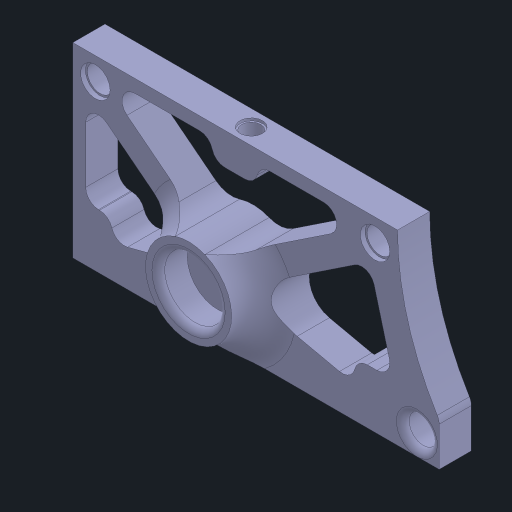
# Autodesk Inventor part: gear_holder_r
Saved by Autodesk Inventor 2023 (Build 270158000, 158)
## iProperties
Created: 2024-06-01
Part Number: gear_holder_r
Material: ABS Plastic
Document SubType Name: Modeling
Designer: szymo
Density: 1.06 g/cm^3
Appearance: Slate Blue
Mass: 5.35805 g
Surface Area: 42.0736 cm^2
Volume: 5.05477 cm^3
TOTAL MASS: 0.0
Author: szymo
Autodesk Inventor part; units mm, degrees
ref_plane "YZ Plane" through (0, 0, 0) normal (1, 0, 0) x (0, 1, 0)
ref_plane "XZ Plane" through (0, 0, 0) normal (0, 1, 0) x (-1, 0, 0)
ref_plane "XY Plane" through (0, 0, 0) normal (0, 0, 1) x (1, 0, 0)
sketch "Sketch10" plane through (0, 0, 0) normal (0, 0, 1) x (1, 0, 0)
  circle A0 centre (29.9359, 0.3357) radius 2 projected
  circle A1 centre (-0.5678, 6.6482) radius 4.5 projected
  circle A2 centre (41.9322, 11.1482) radius 15 projected
  line L0 (99.4322, -2.8518) -> (37.7886, -2.8518) projected
  line L1 (-23.5678, -2.8518) -> (-23.5678, 26.1482) projected
  circle A3 centre (-0.5678, 6.6482) radius 4.575
  circle A4 centre (-0.5678, 6.6482) radius 5.975
  circle A5 centre (29.9359, 0.3357) radius 2.075
  circle A6 centre (29.9359, 0.3357) radius 3.475
  line L2 (22.0831, -2.8518) -> (-23.5678, -2.8518) projected
  line L3 (28.5518, -2.8518) -> (22.0831, -2.8518) projected
  line L4 (31.32, -2.8518) -> (28.5518, -2.8518) projected
  line L5 (37.7886, -2.8518) -> (31.32, -2.8518) projected
  line L6 (-23.5678, 26.1482) -> (111.997, 26.1482) projected
  line L7 (-23.5678, 26.1482) -> (26.9322, 26.1482)
  line L8 (26.9322, 26.1482) -> (26.9322, -2.8518)
  line L9 (26.9322, -2.8518) -> (-23.5678, -2.8518)
  line L10 (-23.5678, -2.8518) -> (-23.5678, 26.1482)
  line L11 (26.9322, 26.1482) -> (19.9322, 26.1482)
  line L12 (19.9322, 26.1482) -> (19.9322, 19.1482)
  line L13 (19.9322, 19.1482) -> (26.9322, 19.1482)
  line L14 (26.9322, 19.1482) -> (26.9322, 26.1482)
  line L15 (-23.5678, 26.1482) -> (-16.5678, 26.1482)
  line L16 (-16.5678, 26.1482) -> (-16.5678, 19.1482)
  line L17 (-16.5678, 19.1482) -> (-23.5678, 19.1482)
  line L18 (-23.5678, 19.1482) -> (-23.5678, 26.1482)
  line L19 (-23.5678, -2.8518) -> (-17.5678, -2.8518)
  line L20 (-17.5678, -2.8518) -> (-17.5678, 5.1482)
  line L21 (-17.5678, 5.1482) -> (-23.5678, 5.1482)
  line L22 (-23.5678, 5.1482) -> (-23.5678, -2.8518)
  line L23 (26.4609, -2.8518) -> (20.4609, -2.8518)
  line L24 (20.4609, -2.8518) -> (20.4609, 5.1482)
  line L25 (20.4609, 5.1482) -> (26.4609, 5.1482)
  line L26 (26.4609, 5.1482) -> (26.4609, -2.8518)
  line L27 (26.9322, -2.8518) -> (33.4109, -2.8518)
  line L28 (33.4109, -2.8518) -> (33.4109, 3.8107)
  line L29 (33.4109, 3.8107) -> (26.9322, 3.8107)
  line L30 (26.9322, 3.8107) -> (26.9322, -2.8518)
  line L31 (26.9322, 26.1482) -> (33.4109, 3.8107)
  circle A7 centre (68.6798, 26.1482) radius 41.7476
  point P0 (0, 0)
  point P1 (28.9333, 3.6629)
  point P2 (28.8494, 3.8107)
  point P3 (29.9359, 3.8107)
  point P4 (38.6488, -2.8518)
  point P5 (26.9322, 26.1482)
  dimension "d122" = 0.075
  dimension "d123" = 1.4
  dimension "d124" = 0.075
  dimension "d125" = 1.4
  dimension "d126" = 7
  dimension "d127" = 7
  dimension "d128" = 7
  dimension "d129" = 7
  dimension "d130" = 6
  dimension "d131" = 8
  dimension "d132" = 6
  dimension "d133" = 8
  constraints: 50 end point, 12 parallel, 6 horizontal, 6 perpendicular, 4 centre point, 4 tangent, 3 point on line, 1 vertical, 3 other
  measures "d122" radial gap between concentric circles of A1 A3
  measures "d123" radial gap between concentric circles of A3 A4
  measures "d124" radial gap between concentric circles of A0 A5
  measures "d125" radial gap between concentric circles of A5 A6
  measures "d126" distance of L13.end L12.end
  measures "d127" distance of L12.end L11.end
  measures "d128" distance of L16.end L17.end
  measures "d129" distance of L15.end L16.end
  measures "d130" distance of L21.end L20.end
  measures "d131" distance of L20.end L19.end
  measures "d132" distance of L24.end L25.end
  measures "d133" distance of L23.end L24.end
extrude "bryla" add sketch "Sketch10" along normal blind 5 contours A0 A2 | A0 A2 A5 | A2 A0 | A0 A2 A5 | A5 A2 A6 L4 L8 | A2 A6 A5 | A6 L8 L29 A2 | A2 L29 A6 | A6 L28 A2 | A2 L28 L5 A6 | L29 L8 A2 | A2 A7 L29 | L29 L28 A6 | L8 A6 | A6 L26 L25 L24 L2 L20 L21 L1 L17 L16 L6 L12 L13 L8 | L8 A7 A2 | L26 L3 L2 L24 L25 | A6 L8 L3 L26 | A6 L3 L8 | L13 L12 L6 L8 | L16 L17 L1 L6 | L2 L1 L21 L20 | A1 | A3 | A4
sketch "Sketch11" plane through (0, 0, 5) normal (0, 0, 1) x (1, 0, 0)
  circle A0 centre (29.9359, 0.3357) radius 2 projected
  arc A1 (29.2892, -11.6469) -> (30.1063, -9.4128) centre (21.6078, -7.5708) ccw projected
  arc A2 (30.1063, -9.4128) -> (30.8013, -9.3758) centre (29.9359, 0.3357) ccw projected
  arc A3 (30.8013, -9.3758) -> (31.851, -11.5105) centre (39.0563, -6.642) ccw projected
  arc A4 (31.851, -11.5105) -> (32.6912, -11.3437) centre (29.9359, 0.3357) ccw projected
  arc A5 (32.6912, -11.3437) -> (32.8459, -8.9699) centre (24.1726, -9.5968) ccw projected
  arc A6 (32.8459, -8.9699) -> (33.5023, -8.7386) centre (29.9359, 0.3357) ccw projected
  arc A7 (33.5023, -8.7386) -> (35.1109, -10.4911) centre (40.6527, -3.7898) ccw projected
  arc A8 (35.1109, -10.4911) -> (35.8701, -10.0943) centre (29.9359, 0.3357) ccw projected
  arc A9 (35.8701, -10.0943) -> (35.3497, -7.7731) centre (27.2044, -10.8182) ccw projected
  arc A10 (35.3497, -7.7731) -> (35.9144, -7.3662) centre (29.9359, 0.3357) ccw projected
  arc A11 (35.9144, -7.3662) -> (37.9515, -8.5945) centre (41.3809, -0.6035) ccw projected
  arc A12 (37.9515, -8.5945) -> (38.5682, -8) centre (29.9359, 0.3357) ccw projected
  arc A13 (38.5682, -8) -> (37.4149, -5.9194) centre (30.4575, -11.1359) ccw projected
  arc A14 (37.4149, -5.9194) -> (37.8421, -5.3699) centre (29.9359, 0.3357) ccw projected
  arc A15 (37.8421, -5.3699) -> (40.1428, -5.9745) centre (41.1819, 2.659) ccw projected
  arc A16 (40.1428, -5.9745) -> (40.5669, -5.2303) centre (29.9359, 0.3357) ccw projected
  arc A17 (40.5669, -5.2303) -> (38.8742, -3.5589) centre (33.6683, -10.5243) ccw projected
  arc A18 (38.8742, -3.5589) -> (39.1293, -2.9114) centre (29.9359, 0.3357) ccw projected
  arc A19 (39.1293, -2.9114) -> (41.5071, -2.8433) centre (40.0718, 5.7333) ccw projected
  arc A20 (41.5071, -2.8433) -> (41.7044, -2.0097) centre (29.9359, 0.3357) ccw projected
  arc A21 (41.7044, -2.0097) -> (39.6094, -0.883) centre (36.5767, -9.0328) ccw projected
  arc A22 (39.6094, -0.883) -> (39.6717, -0.1898) centre (29.9359, 0.3357) ccw projected
  arc A23 (39.6717, -0.1898) -> (41.934, 0.5455) centre (38.1405, 8.3702) ccw projected
  arc A24 (41.934, 0.5455) -> (41.8885, 1.4009) centre (29.9359, 0.3357) ccw projected
  arc A25 (41.8885, 1.4009) -> (39.5609, 1.8918) centre (38.9471, -6.7824) ccw projected
  arc A26 (39.5609, 1.8918) -> (39.4254, 2.5744) centre (29.9359, 0.3357) ccw projected
  arc A27 (39.4254, 2.5744) -> (41.3889, 3.9172) centre (35.5446, 10.3563) ccw projected
  arc A28 (41.3889, 3.9172) -> (41.1043, 4.7252) centre (29.9359, 0.3357) ccw projected
  arc A29 (41.1043, 4.7252) -> (38.7326, 4.5404) centre (40.5875, -3.9553) ccw projected
  arc A30 (38.7326, 4.5404) -> (38.4103, 5.1572) centre (29.9359, 0.3357) ccw projected
  arc A31 (38.4103, 5.1572) -> (39.916, 6.9989) centre (32.4943, 11.5305) ccw projected
  arc A32 (39.916, 6.9989) -> (39.4152, 7.6939) centre (29.9359, 0.3357) ccw projected
  arc A33 (39.4152, 7.6939) -> (37.1917, 6.8484) centre (41.3649, -0.7806) ccw projected
  arc A34 (37.1917, 6.8484) -> (36.7086, 7.3495) centre (29.9359, 0.3357) ccw projected
  arc A35 (36.7086, 7.3495) -> (37.6345, 9.5407) centre (29.2367, 11.7979) ccw projected
  arc A36 (37.6345, 9.5407) -> (36.9582, 10.0664) centre (29.9359, 0.3357) ccw projected
  arc A37 (36.9582, 10.0664) -> (35.063, 8.6288) centre (41.2165, 2.4846) ccw projected
  arc A38 (35.063, 8.6288) -> (34.4583, 8.9734) centre (29.9359, 0.3357) ccw projected
  arc A39 (34.4583, 8.9734) -> (34.7293, 11.3368) centre (26.0358, 11.1366) ccw projected
  arc A40 (34.7293, 11.3368) -> (33.9323, 11.6507) centre (29.9359, 0.3357) ccw projected
  arc A41 (33.9323, 11.6507) -> (32.5188, 9.7373) centre (40.1541, 5.5756) ccw projected
  arc A42 (32.5188, 9.7373) -> (31.8415, 9.8977) centre (29.9359, 0.3357) ccw projected
  arc A43 (31.8415, 9.8977) -> (31.4358, 12.2416) centre (23.1508, 9.6003) ccw projected
  arc A44 (31.4358, 12.2416) -> (30.5826, 12.3183) centre (29.9359, 0.3357) ccw projected
  arc A45 (30.5826, 12.3183) -> (29.7655, 10.0842) centre (38.264, 8.2422) ccw projected
  arc A46 (29.7655, 10.0842) -> (29.0704, 10.0472) centre (29.9359, 0.3357) ccw projected
  arc A47 (29.0704, 10.0472) -> (28.0208, 12.1819) centre (20.8155, 7.3134) ccw projected
  arc A48 (28.0208, 12.1819) -> (27.1805, 12.0151) centre (29.9359, 0.3357) ccw projected
  arc A49 (27.1805, 12.0151) -> (27.0259, 9.6413) centre (35.6991, 10.2682) ccw projected
  arc A50 (27.0259, 9.6413) -> (26.3695, 9.41) centre (29.9359, 0.3357) ccw projected
  arc A51 (26.3695, 9.41) -> (24.7609, 11.1625) centre (19.2191, 4.4613) ccw projected
  arc A52 (24.7609, 11.1625) -> (24.0017, 10.7657) centre (29.9359, 0.3357) ccw projected
  arc A53 (24.0017, 10.7657) -> (24.5221, 8.4445) centre (32.6674, 11.4896) ccw projected
  arc A54 (24.5221, 8.4445) -> (23.9574, 8.0377) centre (29.9359, 0.3357) ccw projected
  arc A55 (23.9574, 8.0377) -> (21.9202, 9.266) centre (18.4909, 1.2749) ccw projected
  arc A56 (21.9202, 9.266) -> (21.3036, 8.6714) centre (29.9359, 0.3357) ccw projected
  arc A57 (21.3036, 8.6714) -> (22.4568, 6.5908) centre (29.4143, 11.8073) ccw projected
  arc A58 (22.4568, 6.5908) -> (22.0297, 6.0413) centre (29.9359, 0.3357) ccw projected
  arc A59 (22.0297, 6.0413) -> (19.729, 6.646) centre (18.6899, -1.9876) ccw projected
  arc A60 (19.729, 6.646) -> (19.3048, 5.9017) centre (29.9359, 0.3357) ccw projected
  arc A61 (19.3048, 5.9017) -> (20.9975, 4.2304) centre (26.2035, 11.1957) ccw projected
  arc A62 (20.9975, 4.2304) -> (20.7425, 3.5828) centre (29.9359, 0.3357) ccw projected
  arc A63 (20.7425, 3.5828) -> (18.3646, 3.5147) centre (19.8, -5.0618) ccw projected
  arc A64 (18.3646, 3.5147) -> (18.1673, 2.6811) centre (29.9359, 0.3357) ccw projected
  arc A65 (18.1673, 2.6811) -> (20.2623, 1.5544) centre (23.2951, 9.7043) ccw projected
  arc A66 (20.2623, 1.5544) -> (20.2001, 0.8612) centre (29.9359, 0.3357) ccw projected
  arc A67 (20.2001, 0.8612) -> (17.9377, 0.126) centre (21.7312, -7.6988) ccw projected
  arc A68 (17.9377, 0.126) -> (17.9832, -0.7294) centre (29.9359, 0.3357) ccw projected
  arc A69 (17.9832, -0.7294) -> (20.3108, -1.2203) centre (20.9247, 7.4538) ccw projected
  arc A70 (20.3108, -1.2203) -> (20.4464, -1.903) centre (29.9359, 0.3357) ccw projected
  arc A71 (20.4464, -1.903) -> (18.4828, -3.2458) centre (24.3272, -9.6849) ccw projected
  arc A72 (18.4828, -3.2458) -> (18.7675, -4.0537) centre (29.9359, 0.3357) ccw projected
  arc A73 (18.7675, -4.0537) -> (21.1391, -3.869) centre (19.2843, 4.6267) ccw projected
  arc A74 (21.1391, -3.869) -> (21.4615, -4.4858) centre (29.9359, 0.3357) ccw projected
  arc A75 (21.4615, -4.4858) -> (19.9558, -6.3274) centre (27.3775, -10.8591) ccw projected
  arc A76 (19.9558, -6.3274) -> (20.4566, -7.0224) centre (29.9359, 0.3357) ccw projected
  arc A77 (20.4566, -7.0224) -> (22.6801, -6.177) centre (18.5068, 1.452) ccw projected
  arc A78 (22.6801, -6.177) -> (23.1631, -6.678) centre (29.9359, 0.3357) ccw projected
  arc A79 (23.1631, -6.678) -> (22.2373, -8.8693) centre (30.6351, -11.1264) ccw projected
  arc A80 (22.2373, -8.8693) -> (22.9136, -9.395) centre (29.9359, 0.3357) ccw projected
  arc A81 (22.9136, -9.395) -> (24.8088, -7.9574) centre (18.6553, -1.8131) ccw projected
  arc A82 (24.8088, -7.9574) -> (25.4135, -8.302) centre (29.9359, 0.3357) ccw projected
  arc A83 (25.4135, -8.302) -> (25.1425, -10.6653) centre (33.836, -10.4652) ccw projected
  arc A84 (25.1425, -10.6653) -> (25.9395, -10.9793) centre (29.9359, 0.3357) ccw projected
  arc A85 (25.9395, -10.9793) -> (27.3529, -9.0659) centre (19.7176, -4.9042) ccw projected
  arc A86 (27.3529, -9.0659) -> (28.0302, -9.2262) centre (29.9359, 0.3357) ccw projected
  arc A87 (28.0302, -9.2262) -> (28.436, -11.5702) centre (36.721, -8.9289) ccw projected
  arc A88 (28.436, -11.5702) -> (29.2892, -11.6469) centre (29.9359, 0.3357) ccw projected
  line L0 (-23.5678, -2.8518) -> (33.4109, -2.8518) projected
  circle A89 centre (29.9359, 0.3357) radius 2.2
  circle A90 centre (29.9359, 0.3357) radius 4.2
  point P0 (0, 0)
  dimension "d136" = 0.2
  dimension "d137" = 2
  constraints: 2 centre point
  measures "d136" radial gap between concentric circles of A0 A89
  measures "d137" radial gap between concentric circles of A89 A90
extrude "smolZebatkaDziura" cut sketch "Sketch11" against normal blind 4 contours A0 | A89
sketch "Sketch12" plane through (0, 0, 5) normal (0, 0, 1) x (1, 0, 0)
  circle A0 centre (-0.5678, 6.6482) radius 4.5 projected
  circle A1 centre (-0.5678, 6.6482) radius 4.7
  point P0 (0, 0)
  dimension "d202" = 0.2
  constraints: 1 centre point
  measures "d202" radial gap between concentric circles of A0 A1
ref_plane "Work Plane4" through (-6.5573, 0.6587, 5.5) normal (0, 0, -1) x (0.4265437, 0.9044669, 0)
extrude "duzaZebatkPodpora" add sketch "Sketch12" along normal up to surface (0.5 mm away) contours A0 | A1
sketch "Sketch13" plane through (0, 0, 5) normal (0, 0, 1) x (1, 0, 0)
  circle A0 centre (-0.5678, 6.6482) radius 4.5 projected
  circle A1 centre (-0.5678, 6.6482) radius 4.7
  circle A2 centre (-0.5678, 6.6482) radius 6.7
  point P0 (0, 0)
  dimension "d142" = 0.2
  dimension "d143" = 2
  constraints: 2 centre point
  measures "d142" radial gap between concentric circles of A0 A1
  measures "d143" radial gap between concentric circles of A1 A2
ref_plane "Work Plane5" through (-6.5573, 0.6587, 8.5) normal (0, 0, 1) x (0.9044669, -0.4265437, 0)
extrude "duzaZebatkaCzymadlo" add sketch "Sketch13" along normal blind 5 contours A2
sketch "Sketch14" plane through (0, 0, 5) normal (0, 0, 1) x (1, 0, 0)
  arc A0 (26.9322, 26.1482) -> (33.4109, 3.8107) centre (68.6798, 26.1482) ccw projected
  line L0 (26.9322, 26.1482) -> (-23.5678, 26.1482) projected
  line L1 (-23.5678, 26.1482) -> (-23.5678, -2.8518) projected
  line L2 (-23.5678, -2.8518) -> (33.4109, -2.8518) projected
  line L3 (33.4109, -2.8518) -> (33.4109, 3.8107) projected
  circle A1 centre (29.9359, 0.3357) radius 2.2 projected
  circle A2 centre (-0.5678, 6.6482) radius 6.7 projected
  line L4 (-23.5678, 26.1482) -> (-16.5678, 26.1482)
  line L5 (-16.5678, 26.1482) -> (-16.5678, 19.1482)
  line L6 (-16.5678, 19.1482) -> (-23.5678, 19.1482)
  line L7 (-23.5678, 19.1482) -> (-23.5678, 26.1482)
  line L8 (-23.5678, -2.8518) -> (-17.5678, -2.8518)
  line L9 (-17.5678, -2.8518) -> (-17.5678, 5.6482)
  line L10 (-17.5678, 5.6482) -> (-23.5678, 5.6482)
  line L11 (-23.5678, 5.6482) -> (-23.5678, -2.8518)
  circle A3 centre (29.9359, 0.3357) radius 3.6
  line L12 (26.3359, -2.8518) -> (20.3359, -2.8518)
  line L13 (20.3359, -2.8518) -> (20.3359, 5.6482)
  line L14 (20.3359, 5.6482) -> (26.3359, 5.6482)
  line L15 (26.3359, 5.6482) -> (26.3359, -2.8518)
  line L16 (26.9322, 26.1482) -> (19.9322, 26.1482)
  line L17 (19.9322, 26.1482) -> (19.9322, 19.1482)
  line L18 (19.9322, 19.1482) -> (26.9322, 19.1482)
  line L19 (26.9322, 19.1482) -> (26.9322, 26.1482)
  line L20 (26.3359, 5.6482) -> (22.7186, 19.1482)
  line L21 (-16.5678, 19.1482) -> (-23.5678, 26.1482) construction
  line L22 (-23.5678, 19.1482) -> (-16.5678, 26.1482) construction
  line L23 (-17.5678, -2.8518) -> (-23.5678, 5.6482) construction
  line L24 (-17.5678, 5.6482) -> (-23.5678, -2.8518) construction
  line L25 (26.3359, -2.8518) -> (20.3359, 5.6482) construction
  line L26 (26.3359, 5.6482) -> (20.3359, -2.8518) construction
  line L27 (19.9322, 19.1482) -> (26.9322, 26.1482) construction
  line L28 (19.9322, 26.1482) -> (26.9322, 19.1482) construction
  line L29 (-16.5678, 19.1482) -> (-0.5678, 6.6482) construction
  line L30 (-0.5678, 6.6482) -> (-20.5678, 1.3982)
  line L31 (-0.5678, 6.6482) -> (23.3359, 1.3982)
  line L32 (-0.5678, 6.6482) -> (23.4322, 22.6482) construction
  line L33 (-17.5678, -0.8518) -> (20.3359, -0.8518)
  line L34 (-21.5678, 5.6482) -> (-21.5678, 19.1482)
  line L35 (-16.5678, 24.1482) -> (19.9322, 24.1482)
  line L36 (-6.8381, 9.0089) -> (-21.5678, 20.5165)
  line L37 (-4.3756, 12.161) -> (-19.7192, 24.1482)
  line L38 (3.6434, 11.8594) -> (22.0767, 24.1482)
  line L39 (22.5775, 19.6747) -> (5.8622, 8.5312)
  point P0 (0, 0)
  point P1 (21.7878, 19.1482)
  point P2 (5.9762, 5.211)
  point P3 (20.3359, 2.0571)
  point P4 (19.9322, 22.7186)
  point P5 (-16.5678, 21.6862)
  point P6 (-19.8164, 19.1482)
  point P7 (-17.5678, 2.1857)
  point P8 (-7.0482, 4.9471)
  dimension "d146" = 7
  dimension "d147" = 7
  dimension "d148" = 6
  dimension "d149" = 8.5
  dimension "d150" = 1.4
  dimension "d151" = 6
  dimension "d152" = 8.5
  dimension "d153" = 7
  dimension "d154" = 7
  dimension "d155" = 0
  dimension "d156" = 0
  dimension "d157" = 75
  dimension "d158" = 0
  dimension "d159" = 0
  dimension "d160" = 2
  dimension "d161" = 2
  dimension "d162" = 2
  dimension "d163" = 2
  dimension "d164" = 2
  dimension "d165" = 2
  dimension "d166" = 2
  constraints: 72 end point, 12 parallel, 12 point on line, 6 perpendicular, 4 horizontal, 4 point on circle, 3 midpoint, 1 centre point, 1 tangent
  measures "d146" distance of L5.end L6.end
  measures "d147" distance of L4.end L5.end
  measures "d148" distance of L10.end L9.end
  measures "d149" distance of L9.end L8.end
  measures "d150" radial gap between concentric circles of A1 A3
  measures "d151" distance of L13.end L14.end
  measures "d152" distance of L12.end L13.end
  measures "d153" distance of L18.end L17.end
  measures "d154" distance of L17.end L16.end
  measures "d155" distance of L0.start L16.start
  measures "d156" distance from line of L0 L16.start
  measures "d157" angle of L18 L20
  measures "d158" distance of L0.start L27.end
  measures "d159" distance of L0.start L27.end
  measures "d160" distance between parallel lines of L0 L35
  measures "d161" distance between parallel lines of L1 L34
  measures "d162" distance between parallel lines of L33 L2
  measures "d163" distance between parallel lines of L38 L32
  measures "d164" distance between parallel lines of L32 L39
  measures "d165" distance between parallel lines of L29 L37
  measures "d166" distance between parallel lines of L29 L36
extrude "zeberka" cut sketch "Sketch14" against normal up to next contours L17 L38 A2 L37 L5 L35 | L20 L14 L13 L31 A2 L39 L18 | L6 L36 A2 L30 L9 L10 L34
sketch "Sketch18" plane through (-23.5678, 26.1482, 0) normal (0, 1, 0) x (1, 0, 0)
  line L0 (50.5, 0) -> (0, 0) projected
  line L1 (0, 0) -> (0, -5) projected
  line L2 (50.5, -5) -> (0, -5) projected
  line L3 (50.5, 0) -> (50.5, -5) projected
  line L4 (7, 0) -> (19.1922, 0) projected
  line L5 (21.75, 0) -> (28.75, 0)
  line L6 (28.75, 0) -> (28.75, -5)
  line L7 (28.75, -5) -> (21.75, -5)
  line L8 (21.75, -5) -> (21.75, 0)
  point P0 (23.5678, 0)
  dimension "d205" = 7
  dimension "d206" = 5
  dimension "d207" = 21.75
  dimension "d208" = 21.75
  constraints: 8 end point, 2 parallel, 1 horizontal, 1 perpendicular, 1 point on line
  measures "d205" distance of L6.end L7.end
  measures "d206" distance of L5.end L6.end
  measures "d207" distance between parallel lines of L1 L8
  measures "d208" distance between parallel lines of L3 L6
extrude "Extrusion12" add sketch "Sketch18" against normal blind 5 contours L6 L2 L8 L0
sketch "Sketch15" plane through (-23.5678, -2.8518, 0) normal (0, -1, 0) x (1, 0, 0)
  line L0 (6, 5) -> (6, 0) projected
  line L1 (43.9037, 5) -> (43.9037, 0) projected
  line L2 (50.5, 0) -> (0, 0) projected
  line L3 (6, 5) -> (0, 5)
  line L4 (0, 5) -> (0, 0)
  line L5 (0, 0) -> (6, 0)
  line L6 (6, 0) -> (6, 5)
  line L7 (43.9037, 5) -> (49.9037, 5)
  line L8 (49.9037, 5) -> (49.9037, 0)
  line L9 (49.9037, 0) -> (43.9037, 0)
  line L10 (43.9037, 0) -> (43.9037, 5)
  line L11 (6, 0) -> (0, 5) construction
  line L12 (0, 0) -> (6, 5) construction
  line L13 (49.9037, 5) -> (43.9037, 0) construction
  line L14 (43.9037, 5) -> (49.9037, 0) construction
  point P0 (23.5678, 0)
  point P1 (3, 2.5)
  point P2 (46.9037, 2.5)
  dimension "d170" = 5
  dimension "d171" = 6
  constraints: 24 end point, 4 parallel, 2 horizontal, 2 midpoint, 2 perpendicular
  measures "d170" distance of L8.end L7.end
  measures "d171" distance between parallel lines of L1 L8
hole "m2.5wPlastik" at (-20.5678, -2.8518, 2.5) at (23.3359, -2.8518, 2.5) direction (0, 1, 0) diameter 2.1 depth 7.99
sketch "Sketch16" plane through (-23.5678, -2.8518, 0) normal (0, -1, 0) x (1, 0, 0)
  circle A0 centre (3, 2.5) radius 1.05 projected
  circle A1 centre (46.9037, 2.5) radius 1.05 projected
  point P0 (23.5678, 0)
  constraints: 2 coincident
hole "m2.5Insert" at (-20.5678, -2.8518, 2.5) at (23.3359, -2.8518, 2.5) direction (0, 1, 0) diameter 3 depth 3 counterbore diameter 3.5 counterbore depth 0.4
sketch "Sketch17" plane through (0, 0, 5) normal (0, 0, 1) x (1, 0, 0)
  circle A0 centre (29.9359, 0.3357) radius 2.2 projected
  arc A1 (26.9322, 26.1482) -> (33.4109, 3.8107) centre (68.6798, 26.1482) ccw projected
  line L0 (26.9322, 26.1482) -> (-23.5678, 26.1482) projected
  line L1 (-23.5678, 26.1482) -> (-23.5678, -2.8518) projected
  line L2 (-23.5678, -2.8518) -> (33.4109, -2.8518) projected
  line L3 (33.4109, -2.8518) -> (33.4109, 3.8107) projected
  line L4 (5.8622, 8.5312) -> (21.7878, 19.1482) projected
  line L5 (21.7878, 19.1482) -> (22.7186, 19.1482) projected
  line L6 (22.7186, 19.1482) -> (26.3359, 5.6482) projected
  line L7 (26.3359, 5.6482) -> (20.3359, 5.6482) projected
  line L8 (20.3359, 5.6482) -> (20.3359, 2.0571) projected
  line L9 (20.3359, 2.0571) -> (5.9762, 5.211) projected
  arc A2 (-7.0482, 4.9471) -> (5.9762, 5.211) centre (-0.5678, 6.6482) ccw projected
  line L10 (-7.0482, 4.9471) -> (-17.5678, 2.1857) projected
  line L11 (-17.5678, 2.1857) -> (-17.5678, 5.6482) projected
  line L12 (-17.5678, 5.6482) -> (-21.5678, 5.6482) projected
  line L13 (-21.5678, 5.6482) -> (-21.5678, 19.1482) projected
  line L14 (-21.5678, 19.1482) -> (-19.8164, 19.1482) projected
  line L15 (-19.8164, 19.1482) -> (-6.8381, 9.0089) projected
  arc A3 (-4.3756, 12.161) -> (-6.8381, 9.0089) centre (-0.5678, 6.6482) ccw projected
  line L16 (-4.3756, 12.161) -> (-16.5678, 21.6862) projected
  line L17 (-16.5678, 21.6862) -> (-16.5678, 24.1482) projected
  line L18 (-16.5678, 24.1482) -> (-1.8178, 24.1482) projected
  line L19 (19.9322, 24.1482) -> (19.9322, 22.7186) projected
  line L20 (19.9322, 22.7186) -> (3.6434, 11.8594) projected
  arc A4 (5.8622, 8.5312) -> (3.6434, 11.8594) centre (-0.5678, 6.6482) ccw projected
  line L21 (-23.5678, 26.1482) -> (-23.5678, -2.8518) projected
  line L22 (-23.5678, 26.1482) -> (-16.5678, 26.1482)
  line L23 (-16.5678, 26.1482) -> (-16.5678, 19.1482)
  line L24 (-16.5678, 19.1482) -> (-23.5678, 19.1482)
  line L25 (-23.5678, 19.1482) -> (-23.5678, 26.1482)
  line L26 (26.9322, 26.1482) -> (19.9322, 26.1482)
  line L27 (19.9322, 26.1482) -> (19.9322, 19.1482)
  line L28 (19.9322, 19.1482) -> (26.9322, 19.1482)
  line L29 (26.9322, 19.1482) -> (26.9322, 26.1482)
  line L30 (-23.5678, 19.1482) -> (-16.5678, 26.1482)
  line L31 (26.9322, 19.1482) -> (19.9322, 26.1482)
  line L32 (19.9322, 19.1482) -> (26.9322, 26.1482)
  line L33 (-16.5678, 19.1482) -> (-23.5678, 26.1482)
  line L34 (5.1822, 24.1482) -> (19.9322, 24.1482) projected
  line L35 (-1.8178, 24.1482) -> (-1.8178, 21.1482) projected
  line L36 (5.1822, 21.1482) -> (-1.8178, 21.1482) projected
  line L37 (5.1822, 24.1482) -> (5.1822, 21.1482) projected
  point P0 (0, 0)
  point P1 (-20.0678, 22.6482)
  point P2 (23.4322, 22.6482)
  dimension "d186" = 7
  dimension "d187" = 7
  dimension "d188" = 7
  dimension "d189" = 7
  dimension "d190" = 0
  dimension "d191" = 0
  constraints: 24 end point, 4 parallel, 2 horizontal, 2 midpoint, 2 perpendicular
  measures "d186" distance of L23.end L24.end
  measures "d187" distance of L22.end L23.end
  measures "d188" distance of L28.end L27.end
  measures "d189" distance of L27.end L26.end
  measures "d190" distance of L0.start L26.start
  measures "d191" distance from line of L0.start L29
hole "m3insert" at (-20.0678, 22.6482, 5) at (23.4322, 22.6482, 5) direction (0, 0, -1) diameter 4 depth 5.75 counterbore diameter 4.6 counterbore depth 0.75
sketch "Sketch19" plane through (-23.5678, 26.1482, 0) normal (0, 1, 0) x (1, 0, 0)
  line L0 (28.75, -5) -> (21.75, -5) projected
  line L1 (21.75, -5) -> (21.75, 0) projected
  line L2 (21.75, 0) -> (28.75, 0) projected
  line L3 (28.75, 0) -> (28.75, -5) projected
  line L4 (28.75, -5) -> (43.5, -5) projected
  line L5 (21.75, 0) -> (28.75, -5)
  line L6 (21.75, -5) -> (28.75, 0)
  point P0 (23.5678, 0)
  point P1 (25.25, -2.5)
  constraints: 4 end point, 1 midpoint
hole "insertUp" at (1.6822, 26.1482, 2.5) direction (0, -1, 0) diameter 3 depth 6 counterbore diameter 3.5 counterbore depth 0.4
fillet "Fillet23" radius 4 6 edges at (-7.0482, 4.9471, 2.5) (-4.3756, 12.161, 2.5) (3.6434, 11.8594, 2.5) (5.8622, 8.5312, 2.5) (5.9762, 5.211, 2.5) (-6.8381, 9.0089, 2.5)
fillet "Fillet19" radius 5 2 edges at (4.9934, 10.385, 5) (-4.511, 1.2315, 5)
fillet "Fillet20" radius 1 2 edges at (27.7359, 0.3357, 5) (-5.2678, 6.6482, 10)
fillet "Fillet21" radius 2 19 edges at (-21.5678, 19.1482, 2.5) (-19.8164, 19.1482, 2.5) (-16.5678, 24.1482, 2.5) (-16.5678, 21.6862, 2.5) (19.9322, 24.1482, 2.5) (19.9322, 22.7186, 2.5) (-17.5678, 2.1857, 2.5) (-17.5678, 5.6482, 2.5) (-21.5678, 5.6482, 2.5) (20.3359, 2.0571, 2.5) (20.3359, 5.6482, 2.5) (26.3359, 5.6482, 2.5) (22.7186, 19.1482, 2.5) (21.7878, 19.1482, 2.5) (33.4109, 3.8107, 2.5) (-1.8178, 24.1482, 2.5) (-1.8178, 21.1482, 2.5) (5.1822, 21.1482, 2.5) (5.1822, 24.1482, 2.5)
body "Solid2"
